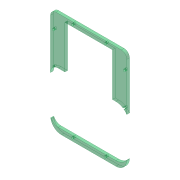
# Autodesk Inventor part: beagle_spacer_top
Saved by Autodesk Inventor 2014 (Build 180170000, 170)
## iProperties
Created: 2013-06-20
Part Number: beagle_spacer_top
Document SubType Name: Modeling
Designer: Administrator
Density: 1 g/cm^3
Mass: 8.38878 g
Surface Area: 71.9101 cm^2
Volume: 8.38878 cm^3
Material: Generic
Appearance: Clear - Green 1
Author: Administrator
Autodesk Inventor part; units mm, degrees
ref_plane "YZ Plane" through (0, 0, 0) normal (1, 0, 0) x (0, 1, 0)
ref_plane "XZ Plane" through (0, 0, 0) normal (0, 1, 0) x (-1, 0, 0)
ref_plane "XY Plane" through (0, 0, 0) normal (0, 0, 1) x (1, 0, 0)
sketch "Sketch1" plane through (0, 0, 0) normal (0, 0, 1) x (1, 0, 0)
  line L0 (9.8795, 48.1994) -> (9.8795, -53.4006)
  line L1 (16.2295, 54.5494) -> (92.4295, 54.5494)
  line L2 (98.7795, 48.1994) -> (98.7795, -53.4006)
  line L3 (22.5795, -66.1006) -> (86.0795, -66.1006)
  arc A0 (9.8795, -53.4006) -> (22.5795, -66.1006) centre (22.5795, -53.4006) ccw
  arc A1 (16.2295, 54.5494) -> (9.8795, 48.1994) centre (16.2295, 48.1994) ccw
  arc A2 (98.7795, 48.1994) -> (92.4295, 54.5494) centre (92.4295, 48.1994) ccw
  arc A3 (86.0795, -66.1006) -> (98.7795, -53.4006) centre (86.0795, -53.4006) ccw
  point P0 (0, 0)
  dimension "d0" = 12.7
  dimension "d1" = 6.35
  dimension "d2" = 120.65
  dimension "d3" = 88.9
  constraints: 8 end point, 8 point on circle, 8 tangent, 4 centre point, 2 equal radius, 1 horizontal, 1 vertical
  measures "d0" radius of A0
  measures "d1" radius of A1
  measures "d2" distance between parallel lines of L3 L1
  measures "d3" distance between parallel lines of L2 L0
extrude "Extrusion1" add sketch "Sketch1" along normal blind 3.175
sketch "Sketch2" plane through (0, 0, 3.175) normal (0, 0, 1) x (1, 0, 0)
  line L0 (9.8795, -53.4006) -> (9.8795, 48.1994) projected
  line L1 (98.7795, 48.1994) -> (98.7795, -53.4006) projected
  line L2 (16.2295, 54.5494) -> (92.4295, 54.5494) projected
  line L3 (26.6435, 49.4694) -> (82.0155, 49.4694)
  line L4 (82.0155, 49.4694) -> (82.0155, -1.3306)
  line L5 (82.0155, -1.3306) -> (26.6435, -1.3306)
  line L6 (26.6435, -1.3306) -> (26.6435, 49.4694)
  point P0 (0, 0)
  dimension "d13" = 16.764
  dimension "d14" = 16.764
  dimension "d15" = 5.08
  dimension "d16" = 55.88
  constraints: 8 end point
  measures "d13" distance between parallel lines of L0 L6
  measures "d14" distance between parallel lines of L1 L4
  measures "d15" distance between parallel lines of L2 L3
  measures "d16" distance between parallel lines of L5 L2
extrude "Extrusion2" cut sketch "Sketch2" against normal through all
sketch "Sketch8" plane through (0, 0, 3.175) normal (0, 0, 1) x (1, 0, 0)
  line L0 (82.0155, -1.3306) -> (26.6435, -1.3306) projected
  line L1 (9.8795, -53.4006) -> (9.8795, 48.1994) projected
  line L2 (98.7795, 48.1994) -> (98.7795, -53.4006) projected
  line L3 (18.7695, -2.6006) -> (86.0795, -2.6006)
  line L4 (12.3173, -6.9948) -> (9.8795, -6.9948)
  arc A0 (86.1117, -10.6693) -> (86.0795, -10.656) centre (83.9402, -15.8848) ccw
  line L5 (86.0795, -66.1006) -> (22.5795, -66.1006) projected
  arc A1 (18.7695, -2.6006) -> (12.3173, -6.9948) centre (18.7695, -9.5348) ccw
  arc A2 (9.8795, -51.4448) -> (18.7695, -60.3348) centre (18.7695, -51.4448) ccw
  arc A3 (86.0795, -60.3348) -> (98.7795, -53.519) centre (86.0795, -45.0948) ccw
  line L6 (86.0795, -60.3348) -> (18.7695, -60.3348)
  arc A4 (98.7795, -15.3006) -> (86.0795, -2.6006) centre (86.0795, -15.3006) ccw
  line L7 (9.8795, -6.9948) -> (9.8795, -51.4448)
  line L8 (98.7795, -15.3006) -> (98.7795, -53.519)
  point P0 (0, 0)
  dimension "d70" = 1.27
  dimension "d89" = 8.89
  dimension "d90" = 56.5658
  dimension "d95" = 8.89
  dimension "d96" = 14.6558
  dimension "d101" = 12.7
  dimension "d102" = 21.0058
  dimension "d103" = 12.7
  dimension "d104" = 50.2158
  dimension "d105" = 5.7658
  dimension "d107" = 59.1058
  constraints: 10 end point, 10 point on circle, 5 centre point, 5 tangent, 4 point on line, 2 horizontal
  measures "d70" distance between parallel lines of L0 L3
  measures "d89" distance from line of L1 A1.centre
  measures "d90" distance from line of L5 A1.centre
  measures "d95" distance from line of L1 A2.centre
  measures "d96" distance from line of L5 A2.centre
  measures "d101" distance from line of L2 A3.centre
  measures "d102" distance from line of L5 A3.centre
  measures "d103" distance from line of L2 A4.centre
  measures "d104" distance from line of L5 A0.centre
  measures "d105" distance between parallel lines of L5 L6
  measures "d107" distance between parallel lines of L5 L4
extrude "Extrusion16" [suppressed]
sketch "Sketch9" plane through (0, 0, 3.175) normal (0, 0, 1) x (1, 0, 0)
  line L0 (9.8795, -53.4006) -> (9.8795, 48.1994) projected
  line L1 (86.0795, -66.1006) -> (22.5795, -66.1006) projected
  line L2 (98.7795, 48.1994) -> (98.7795, -53.4006) projected
  arc A0 (18.7695, -3.1848) -> (12.4195, -9.5348) centre (18.7695, -9.5348) ccw
  arc A1 (98.7795, -15.8848) -> (86.0795, -3.1848) centre (86.0795, -15.8848) ccw
  arc A2 (12.4195, -51.4448) -> (18.7695, -57.7948) centre (18.7695, -51.4448) ccw
  arc A3 (86.0795, -57.7948) -> (98.7795, -45.0948) centre (86.0795, -45.0948) ccw
  line L3 (18.7695, -3.1848) -> (86.0795, -3.1848)
  line L4 (98.7795, -15.8848) -> (98.7795, -45.0948)
  line L5 (86.0795, -57.7948) -> (18.7695, -57.7948)
  line L6 (12.4195, -51.4448) -> (12.4195, -9.5348)
  arc A4 (101.3195, -15.8848) -> (86.0795, -0.6448) centre (86.0795, -15.8848) ccw
  line L7 (101.3195, -15.8848) -> (101.3195, -45.0948)
  arc A5 (86.0795, -60.3348) -> (101.3195, -45.0948) centre (86.0795, -45.0948) ccw
  line L8 (86.0795, -60.3348) -> (18.7695, -60.3348)
  arc A6 (9.8795, -51.4448) -> (18.7695, -60.3348) centre (18.7695, -51.4448) ccw
  line L9 (9.8795, -51.4448) -> (9.8795, -9.5348)
  arc A7 (18.7695, -0.6448) -> (9.8795, -9.5348) centre (18.7695, -9.5348) ccw
  line L10 (18.7695, -0.6448) -> (86.0795, -0.6448)
  point P0 (0, 0)
  dimension "d110" = 6.35
  dimension "d111" = 6.35
  dimension "d112" = 12.7
  dimension "d113" = 12.7
  dimension "d114" = 54.61
  dimension "d115" = 86.36
  dimension "d116" = 8.3058
  constraints: 16 end point, 16 point on circle, 8 centre point, 8 tangent, 2 collinear, 2 horizontal, 2 vertical, 7 other
  measures "d110" radius of A0
  measures "d111" radius of A2
  measures "d112" radius of A3
  measures "d113" radius of A1
  measures "d114" distance between parallel lines of L5 L3
  measures "d115" distance between parallel lines of L4 L6
  measures "d116" distance between parallel lines of L1 L5
extrude "Extrusion17" cut sketch "Sketch9" against normal through all contours L2 A3 L5 A2 L6 A0 L3 A1 | L0 A7 L10 A4 L7 A5 L8 A6
sketch "Sketch10" plane through (0, 0, 3.175) normal (0, 0, 1) x (1, 0, 0)
  arc A0 (9.8795, -51.4448) -> (18.7695, -60.3348) centre (18.7695, -51.4448) ccw projected
  line L0 (9.8795, -53.4006) -> (9.8795, -51.4448) projected
  arc A1 (9.8795, -53.4006) -> (22.5795, -66.1006) centre (22.5795, -53.4006) ccw projected
  line L1 (10.0156, -55.2548) -> (10.7373, -55.2548)
  point P0 (0, 0)
  dimension "d119" = 3.81
  constraints: 2 end point, 2 point on circle, 1 horizontal
  measures "d119" distance from line of L0.end L1
extrude "Extrusion18" cut sketch "Sketch10" against normal through all
sketch "Sketch11" plane through (0, 0, 3.175) normal (0, 0, 1) x (1, 0, 0)
  line L0 (98.7795, 48.1994) -> (98.7795, -7.4606) projected
  line L1 (16.2295, 54.5494) -> (92.4295, 54.5494) projected
  line L2 (9.8795, -9.5348) -> (9.8795, 48.1994) projected
  circle A0 centre (13.0037, 35.4994) radius 1.27
  circle A1 centre (13.0037, -2.6006) radius 1.27
  circle A2 centre (35.2795, 51.4252) radius 1.27
  circle A3 centre (73.3795, 51.4252) radius 1.27
  circle A4 centre (95.6553, 35.4994) radius 1.27
  circle A5 centre (95.6553, -2.6006) radius 1.27
  circle A6 centre (73.3795, -62.9764) radius 1.27
  circle A7 centre (35.2795, -62.9764) radius 1.27
  line L3 (86.0795, -66.1006) -> (22.5795, -66.1006) projected
  point P0 (0, 0)
  dimension "d122" = 3.1242
  dimension "d123" = 3.1242
  dimension "d124" = 3.1242
  dimension "d125" = 2.54
  dimension "d126" = 19.05
  dimension "d127" = 3.1242
  dimension "d129" = 38.1
  dimension "d130" = 25.4
  dimension "d131" = 38.1
  constraints: 8 centre point, 7 equal radius, 4 horizontal alignment, 4 vertical alignment
  measures "d122" distance from line of L3 A7.centre
  measures "d123" distance from line of L2 A0.centre
  measures "d124" distance from line of L1 A2.centre
  measures "d125" diameter of A2
  measures "d126" distance from line of L1 A0.centre
  measures "d127" distance from line of L0 A4.centre
  measures "d129" distance of A3.centre A2.centre
  measures "d130" distance from line of L2 A2.centre
  measures "d131" distance of A1.centre A0.centre
extrude "Extrusion19" cut sketch "Sketch11" against normal through all
equation "\"d14\" = d13"
body "Solid1"
